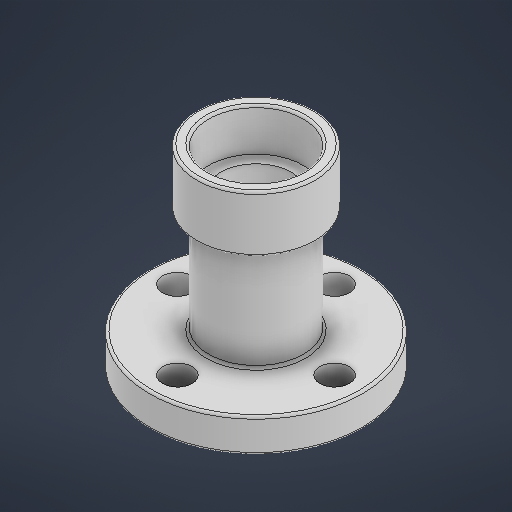
# Autodesk Inventor part: b9
Saved by Autodesk Inventor 2025.4 (Build 294407000, 407)
## iProperties
Created: 2026-05-07
Part Number: b9
Material: Generic
Document SubType Name: Modeling
Designer: VuQuan
Density: 1 g/cm^3
Appearance: Default
Author: VuQuan
Autodesk Inventor part; units mm, degrees
ref_plane "YZ Plane" through (0, 0, 0) normal (1, 0, 0) x (0, 1, 0)
ref_plane "XZ Plane" through (0, 0, 0) normal (0, 1, 0) x (-1, 0, 0)
ref_plane "XY Plane" through (0, 0, 0) normal (0, 0, 1) x (1, 0, 0)
sketch "Sketch1" plane through (0, 0, 0) normal (0, 0, 1) x (1, 0, 0)
  line L0 (0, 0) -> (0, 82.4) construction
  line L1 (18, 0) -> (45, 0)
  line L2 (45, 0) -> (45, 14.2)
  line L3 (45, 14.2) -> (20, 14.2)
  line L4 (20, 14.2) -> (20, 58.4)
  line L5 (20, 58.4) -> (25, 58.4)
  line L6 (25, 58.4) -> (25, 82.4)
  line L7 (25, 82.4) -> (20, 82.4)
  line L8 (20, 82.4) -> (20, 64.4)
  line L9 (20, 64.4) -> (15, 64.4)
  line L10 (15, 64.4) -> (15, 3.5)
  line L11 (15, 3.5) -> (18, 0)
  point P0 (15, 0)
  dimension "d0" = 40
  dimension "d1" = 90
  dimension "d2" = 50
  dimension "d3" = 18
  dimension "d4" = 6
  dimension "d5" = 44.2
  dimension "d6" = 14.2
  dimension "d7" = 3.5
  dimension "d8" = 3
  constraints: 24 end point, 8 perpendicular, 3 point on line, 2 horizontal, 1 collinear, 1 horizontal alignment, 1 parallel, 1 vertical
  measures "d0" diameter of L8 L0
  measures "d1" diameter of L2 L0
  measures "d2" diameter of L6 L0
  measures "d3" distance between parallel lines of L7 L9
  measures "d4" distance between parallel lines of L9 L5
  measures "d5" distance between parallel lines of L5 L3
  measures "d6" distance of L1.end L2.end
  measures "d7" distance of L10.end point (15, 0)
  measures "d8" distance of L1.start point (15, 0)
revolve "Revolution1" add sketch "Sketch1" angle 360 about axis through (0, 0, 0) along (0, 1, 0)
fillet "Fillet1" radius 1 7 edges at (-25, 82.4, 0) (-20, 82.4, 0) (-25, 58.4, 0) (-20, 58.4, 0) (-20, 14.2, 0) (-45, 14.2, 0) (-45, 0, 0)
sketch "Sketch2" plane through (0, 14.2, 0) normal (0, 1, 0) x (1, 0, 0)
  circle A0 centre (0, 0) radius 21 projected
  circle A1 centre (33.25, 0) radius 6.25
  dimension "d11" = 12.5
  dimension "d12" = 33.25
  constraints: 1 centre point, 1 horizontal alignment
  measures "d11" diameter of A1
  measures "d12" distance of A0.centre A1.centre
extrude "Extrusion1" cut sketch "Sketch2" against normal through all contours A1
pattern_circular "Circular Pattern1" count 4 over 360 about axis through (0, 33.95, 0) along (0, 1, 0) of "Extrusion1"
body "Solid1"
